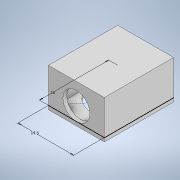
# Autodesk Inventor part: carcasaXeotype_BUZZER
Saved by Autodesk Inventor 2020 (Build 240168000, 168)
## iProperties
Created: 2021-04-10
Part Number: carcasaXeotype_BUZZER
Material: Generic
Document SubType Name: Modeling
Designer: Vlasciar
Density: 1 g/cm^3
Appearance: Default
Author: Vlasciar
Autodesk Inventor part; units mm, degrees
ref_plane "YZ Plane" through (0, 0, 0) normal (1, 0, 0) x (0, 1, 0)
ref_plane "XZ Plane" through (0, 0, 0) normal (0, 1, 0) x (-1, 0, 0)
ref_plane "XY Plane" through (0, 0, 0) normal (0, 0, 1) x (1, 0, 0)
sketch "Sketch1" plane through (0, 0, 0) normal (0, 1, 0) x (-1, 0, 0)
  line L0 (-7.25, -9) -> (7.25, -9)
  line L1 (7.25, -9) -> (7.25, 9)
  line L2 (7.25, 9) -> (-7.25, 9)
  line L3 (-7.25, 9) -> (-7.25, -9)
  line L4 (-7.25, -9) -> (7.25, 9) construction
  line L5 (7.25, -9) -> (-7.25, 9) construction
  point P0 (0, 0)
  dimension "d0" = 14.5
  dimension "d1" = 18
  constraints: 12 end point, 2 midpoint, 2 parallel, 1 horizontal, 1 perpendicular
  measures "d0" distance of L1.end L2.end
  measures "d1" distance of L0.end L1.end
extrude "Extrusion1" add sketch "Sketch1" along normal blind 8 and the other way blind 1
sketch "Sketch2" plane through (0, -1, 0) normal (0, -1, 0) x (1, 0, 0)
  line L0 (-7.25, 9) -> (-7.25, -9) projected
  line L1 (-7.25, -9) -> (7.25, -9) projected
  circle A0 centre (0, -1.25) radius 6.25
  point P0 (0, 0)
  dimension "d7" = 1.5
  dimension "d8" = 1
  dimension "d9" = 12.5
  constraints: 1 centre point, 1 vertical alignment
  measures "d7" distance edge to line of A0 L1
  measures "d8" distance edge to line of A0 L0
  measures "d9" diameter of A0
extrude "Extrusion2" cut sketch "Sketch2" against normal blind 8
sketch "Sketch3" plane through (-7.25, 8, 9) normal (0, 0, 1) x (1, 0, 0)
  line L0 (0, 0) -> (14.5, 0) projected
  circle A0 centre (7.25, -4.5) radius 3.5
  point P0 (7.25, -8)
  dimension "d14" = 1
  constraints: 1 centre point
  measures "d14" distance edge to line of A0 L0
extrude "Extrusion3" cut sketch "Sketch3" against normal blind 8
sketch "Sketch4" plane through (0, 8, 0) normal (0, 1, 0) x (1, 0, 0)
  line L0 (-7.25, 9) -> (-7.25, -9) projected
  line L1 (-7.25, -9) -> (7.25, -9) projected
  line L2 (7.25, -9) -> (7.25, 9) projected
  line L3 (7.25, 9) -> (-7.25, 9) projected
  line L4 (6.25, -8) -> (-6.25, -8)
  line L5 (-6.25, -8) -> (-6.25, 8)
  line L6 (-6.25, 8) -> (6.25, 8)
  line L7 (6.25, 8) -> (6.25, -8)
  point P0 (0, 0)
  dimension "d17" = 1
  dimension "d18" = 1
  dimension "d19" = 1
  dimension "d20" = 1
  constraints: 8 end point, 2 parallel, 1 horizontal, 1 perpendicular
  measures "d17" distance between parallel lines of L1 L4
  measures "d18" distance between parallel lines of L2 L7
  measures "d19" distance between parallel lines of L0 L5
  measures "d20" distance between parallel lines of L3 L6
extrude "Extrusion4" cut sketch "Sketch4" against normal blind 8 contours L4 L5 L6 L7
sketch "Sketch5" plane through (0, 8, 0) normal (0, 1, 0) x (1, 0, 0)
  line L0 (-7.25, 9) -> (-7.25, -9) projected
  line L1 (-7.25, -9) -> (7.25, -9) projected
  line L2 (7.25, -9) -> (7.25, 9) projected
  line L3 (7.25, 9) -> (-7.25, 9) projected
  line L4 (7.25, -9) -> (-7.25, -9) projected
  line L5 (7.25, 9) -> (-7.25, 9)
  line L6 (-7.25, 9) -> (-7.25, -9)
  line L7 (-7.25, -9) -> (7.25, -9)
  line L8 (7.25, -9) -> (7.25, 9)
  point P0 (0, 0)
  constraints: 8 end point, 2 parallel, 1 horizontal, 1 perpendicular
extrude "Extrusion5" add sketch "Sketch5" along normal blind 1
body "Solid1"
